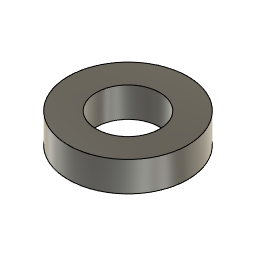
Question 4 Assembly (Autodesk Fusion 360 archive; units mm, degrees)
design "Spacer"
Autodesk Fusion 360 part; units mm, degrees
sketch "Sketch1" plane through (0, 0, 0) normal (0, 0, 1) x (1, 0, 0)
  circle A0 centre (0, 0) radius 8
  circle A1 centre (0, 0) radius 4.25
  dimension "d1" = 16
  dimension "d2" = 8.5
  constraint coincident A0.centre A1.centre
  measures "d1" diameter of A0
  measures "d2" diameter of A1
extrude "Extrude1" add sketch "Sketch1" along normal blind 4 makes body 1
copy_body "Body->Comp1" bodies 1 removing the originals makes body 2 in component "Component"
component "Component" placed x (1, 0, 0) y (0, 1, 0) z (0, 0, 1) at (0, 0, 0)

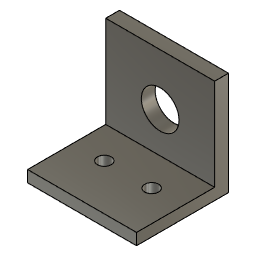
design "Support"
Autodesk Fusion 360 part; units mm, degrees
sketch "Sketch1" plane through (0, 0, 0) normal (0, 0, 1) x (1, 0, 0)
  line L0 (0, 0) -> (23.7, 0)
  line L1 (23.7, 0) -> (23.7, 20)
  line L2 (23.7, 20) -> (0, 20)
  line L3 (0, 20) -> (0, 0)
  line L4 (17, 0) -> (17, 10)
  circle A0 centre (17, 10) radius 1.5
  circle A1 centre (6.7, 10) radius 1.5
  dimension "d1" = 23.7
  dimension "d2" = 20
  dimension "d3" = 10
  dimension "d4" = 6.7
  dimension "d5" = 3
  dimension "d8" = -10.3
  dimension "d9" = 0
  constraint coincident L0.start L3.end
  constraint horizontal L0
  constraint perpendicular L0 L1
  constraint perpendicular L1 L2
  constraint perpendicular L0 L3
  constraint coincident L0 L4.start
  constraint perpendicular L0 L4
  constraint coincident L4.end A0.centre
  measures "d1" distance of L0.start L0.end
  measures "d2" distance of L0.end L1.end
  measures "d3" distance of L4.start L4.end
  measures "d4" distance of L1 L4
  measures "d5" diameter of A0
extrude "Extrude1" add sketch "Sketch1" along normal blind 2.5 makes body 1
sketch "Sketch2" plane through (0, 0, 2.5) normal (0, 0, 1) x (-1, 0, 0)
  circle A0 centre (-6.7, -10) radius 1.5
  circle A1 centre (-17, -10) radius 1.5
  line L0 (0, -20) -> (0, 0)
  line L1 (0, 0) -> (-23.7, 0)
  line L2 (-23.7, 0) -> (-23.7, -20)
  line L3 (-23.7, -20) -> (0, -20)
  line L4 (-23.7, -20) -> (-23.7, -17)
  line L5 (-23.7, -17) -> (0, -17)
  dimension "d12" = 3
  constraint coincident L2.end L3.start
  constraint perpendicular L3 L4
  constraint coincident L0 L5.end
  constraint perpendicular L0 L5
  measures "d12" distance of L2.end L4.end
extrude "Extrude2" add sketch "Sketch2" along normal blind 20 contours L0 L2 L3 L4 L5 bodies 1
sketch "Sketch3" plane through (0, 20, 0) normal (0, 1, 0) x (-1, 0, 0)
  line L0 (-23.7, 0) -> (0, 0)
  line L1 (0, 0) -> (0, 22.5)
  line L2 (0, 22.5) -> (-23.7, 22.5)
  line L3 (-23.7, 22.5) -> (-23.7, 0)
  line L4 (-23.7, 22.5) -> (0, 0)
  circle A0 centre (-11.85, 11.25) radius 4.1
  dimension "d15" = 8.2
  constraint coincident L2.end L3.start
  constraint coincident L0.end L1.start
  constraint midpoint L4 A0.centre
  measures "d15" diameter of A0
extrude "Extrude3" cut sketch "Sketch3" against normal blind 3 contours L4 A0 | L4 A0 bodies 1
copy_body "Body->Comp1" bodies 1 removing the originals makes body 2 in component "Component"
component "Component" placed x (1, 0, 0) y (0, 1, 0) z (0, 0, 1) at (0, 0, 0)

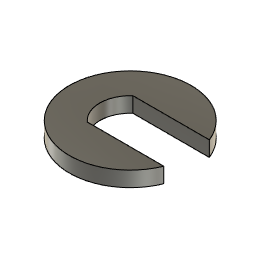
design "Collar"
Autodesk Fusion 360 part; units mm, degrees
sketch "Sketch1" plane through (0, 0, 0) normal (0, 0, 1) x (1, 0, 0)
  circle A0 centre (0, 0) radius 8
  circle A1 centre (0, 0) radius 4
  line L0 (11, -3) -> (-11, -3)
  line L1 (-11, -3) -> (-11, 3)
  line L2 (-11, 3) -> (11, 3)
  line L3 (11, 3) -> (11, -3)
  line L4 (11, -3) -> (-11, 3) construction
  line L5 (-11, -3) -> (11, 3) construction
  dimension "d1" = 16
  dimension "d2" = 8
  constraint coincident A0.centre A1.centre
  constraint horizontal L0
  constraint perpendicular L0 L1
  constraint parallel L0 L2
  constraint parallel L1 L3
  constraint coincident L4 A0.centre
  constraint coincident L5 A0.centre
  measures "d1" diameter of A0
  measures "d2" diameter of A1
extrude "Extrude1" add sketch "Sketch1" along normal blind 2 contours A0 A1 L2 | A0 A1 L0 | A0 A1 L0 L2 | A1 L2 | A1 L0 picked at (-6.3321, 2.0478) makes body 1
copy_body "Body->Comp1" bodies 1 removing the originals makes body 2 in component "Component"
component "Component" placed x (1, 0, 0) y (0, 1, 0) z (0, 0, 1) at (0, 0, 0)

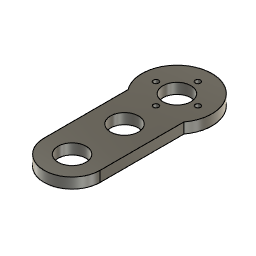
design "Input_Link"
Autodesk Fusion 360 part; units mm, degrees
sketch "Sketch1" plane through (0, 0, 0) normal (0, 0, 1) x (1, 0, 0)
  circle A0 centre (0, 0) radius 10
  circle A1 centre (0, 0) radius 4
  circle A2 centre (0, -15) radius 4
  circle A3 centre (0, -30) radius 4
  circle A4 centre (0, -30) radius 8
  line L0 (-8, -6) -> (-8, -30)
  line L1 (8, -6) -> (8, -30)
  line L2 (0, 0) -> (6, 0)
  circle A5 centre (6, 0) radius 0.75
  circle A6 centre (0, 6) radius 0.75
  circle A7 centre (-6, 0) radius 0.75
  circle A8 centre (0, -6) radius 0.75
  dimension "d1" = 20
  dimension "d2" = 8
  dimension "d5" = 0
  dimension "d6" = -30
  dimension "d7" = 16
  dimension "d9" = 8
  dimension "d12" = 6
  dimension "d14" = 360
  dimension "d15" = 1.5
  dimension "d16" = 8
  constraint coincident A0.centre A1.centre
  constraint concentric A3 A4
  constraint coincident A4 L0.end
  constraint coincident A0 L0.start
  constraint coincident A4 L1.end
  constraint coincident A0 L1.start
  constraint horizontal L2
  constraint coincident L2.end A5.centre
  measures "d1" diameter of A0
  measures "d2" diameter of A1
  measures "d7" diameter of A4
  measures "d9" distance of A3.centre L0
  measures "d12" distance of A0.centre L2.end
  measures "d15" diameter of A5
  measures "d16" distance of A3.centre L1
extrude "Extrude1" add sketch "Sketch1" along normal blind 3 makes body 1
copy_body "Body->Comp1" bodies 1 removing the originals makes body 2 in component "Component"
component "Component" placed x (1, 0, 0) y (0, 1, 0) z (0, 0, 1) at (0, 0, 0)

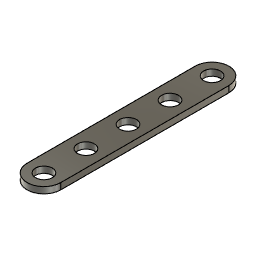
design "Coupler_Link"
Autodesk Fusion 360 part; units mm, degrees
sketch "Sketch1" plane through (0, 0, 0) normal (0, 0, 1) x (1, 0, 0)
  circle A0 centre (0, 0) radius 4
  circle A1 centre (0, 0) radius 8
  line L0 (-8, 0) -> (-8, -80)
  line L1 (8, 0) -> (8, -80)
  circle A2 centre (0, -80) radius 8
  circle A3 centre (0, -20) radius 4
  circle A4 centre (0, -40) radius 4
  circle A5 centre (0, -60) radius 4
  circle A6 centre (0, -80) radius 4
  dimension "d1" = 8
  dimension "d2" = 16
  dimension "d3" = 80
  dimension "d4" = 80
  dimension "d7" = 0
  dimension "d8" = -80
  dimension "d9" = 80
  dimension "d10" = 16
  constraint coincident A0.centre A1.centre
  constraint concentric A0 A1
  constraint coincident A1 L0.start
  constraint vertical L0
  constraint coincident A1 L1.start
  constraint coincident L1.end A2
  measures "d1" diameter of A0
  measures "d2" diameter of A1
  measures "d3" distance of L0.start L0.end
  measures "d4" distance of L1.start L1.end
  measures "d9" distance of A0.centre A2.centre
  measures "d10" distance of L0 L1
extrude "Extrude1" add sketch "Sketch1" along normal blind 3 makes body 1
copy_body "Body->Comp1" bodies 1 removing the originals makes body 2 in component "Component"
component "Component" placed x (1, 0, 0) y (0, 1, 0) z (0, 0, 1) at (0, 0, 0)

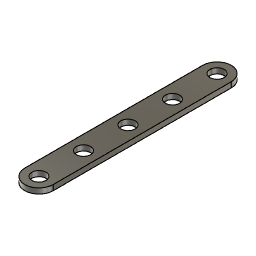
design "Output_Link"
Autodesk Fusion 360 part; units mm, degrees
sketch "Sketch1" plane through (0, 0, 0) normal (0, 0, 1) x (1, 0, 0)
  circle A0 centre (0, 0) radius 4
  circle A1 centre (0, 0) radius 8
  line L0 (-8, 0) -> (-8, -100)
  line L1 (8, 0) -> (8, -100)
  circle A2 centre (0, -100) radius 8
  circle A3 centre (0, -25) radius 4
  circle A4 centre (0, -50) radius 4
  circle A5 centre (0, -75) radius 4
  circle A6 centre (0, -100) radius 4
  dimension "d1" = 8
  dimension "d2" = 16
  dimension "d3" = 100
  dimension "d4" = 100
  dimension "d7" = 0
  dimension "d8" = -100
  constraint coincident A0.centre A1.centre
  constraint coincident A1 L0.start
  constraint tangent A1 L0
  constraint coincident A1 L1.start
  constraint coincident L1.end A2
  measures "d1" diameter of A0
  measures "d2" diameter of A1
  measures "d3" distance of L0.start L0.end
  measures "d4" distance of L1.start L1.end
extrude "Extrude1" add sketch "Sketch1" along normal blind 3 makes body 1
copy_body "Body->Comp1" bodies 1 removing the originals makes body 2 in component "Component"
component "Component" placed x (1, 0, 0) y (0, 1, 0) z (0, 0, 1) at (0, 0, 0)

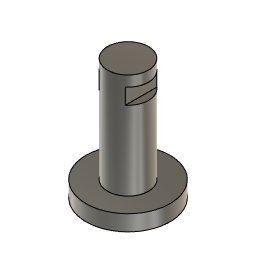
design "Pin_Joint"
Autodesk Fusion 360 part; units mm, degrees
sketch "Sketch1" plane through (0, 0, 0) normal (0, 0, 1) x (1, 0, 0)
  circle A0 centre (0, 0) radius 8
  dimension "d1" = 16
  constraint coincident A0.centre origin
  measures "d1" diameter of A0
extrude "Extrude1" add sketch "Sketch1" along normal blind 3 makes body 1
sketch "Sketch2" plane through (0, 0, 3) normal (0, 0, 1) x (-1, 0, 0)
  circle A0 centre (0, 0) radius 8
  circle A1 centre (0, 0) radius 3.9
  dimension "d4" = 7.8
  constraint concentric A0 A1
  measures "d4" diameter of A1
extrude "Extrude2" add sketch "Sketch2" along normal blind 15 contours A1 bodies 1
sketch "Sketch3" plane through (0, 0, 18) normal (0, 0, 1) x (-1, 0, 0)
  circle A0 centre (0, 0) radius 3.9
  line L0 (-2.5, -6.25) -> (2.5, -6.25)
  line L1 (2.5, -6.25) -> (2.5, 6.25)
  line L2 (2.5, 6.25) -> (-2.5, 6.25)
  line L3 (-2.5, 6.25) -> (-2.5, -6.25)
  line L4 (-2.5, -6.25) -> (2.5, 6.25) construction
  line L5 (2.5, -6.25) -> (-2.5, 6.25) construction
  dimension "d12" = 5
  constraint horizontal L0
  constraint perpendicular L0 L1
  constraint parallel L0 L2
  constraint parallel L1 L3
  constraint coincident L4 A0.centre
  constraint coincident L5 A0.centre
  constraint coincident A0.centre origin
  measures "d12" distance of L1 L3
extrude "Extrude3" add sketch "Sketch3" along normal blind 3 contours A0 L1 L3 bodies 1
sketch "Sketch4" plane through (0, 0, 21) normal (0, 0, 1) x (-1, 0, 0)
  arc A0 (2.5, 2.9933) -> (-2.5, 2.9933) centre (0, 0) ccw
  line L0 (-2.5, 2.9933) -> (-2.5, -2.9933)
  arc A1 (-2.5, -2.9933) -> (2.5, -2.9933) centre (0, 0) ccw
  line L1 (2.5, -2.9933) -> (2.5, 2.9933)
  circle A2 centre (0, 0) radius 3.9
  dimension "d9" = 7.8
  constraint concentric A0 A2
  measures "d9" diameter of A2
extrude "Extrude4" add sketch "Sketch4" along normal blind 2 bodies 1
copy_body "Body->Comp1" bodies 1 removing the originals makes body 2 in component "Component"
component "Component" placed x (1, 0, 0) y (0, 1, 0) z (0, 0, 1) at (0, 0, 0)

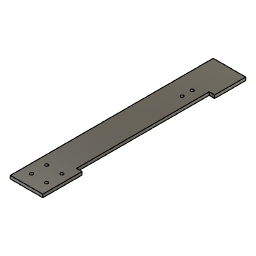
design "Base_Link"
Autodesk Fusion 360 part; units mm, degrees
sketch "Sketch3" plane through (0, 0, 0) normal (0, 0, 1) x (1, 0, 0)
  line L0 (0, 0) -> (0, 200)
  line L1 (0, 200) -> (32.04, 200)
  line L2 (32.04, 200) -> (32.04, 169.36)
  line L3 (32.04, 169.36) -> (26.64, 169.36)
  line L4 (0, 0) -> (32.04, 0)
  line L5 (32.04, 0) -> (32.04, 38.69)
  line L6 (32.04, 38.69) -> (26.64, 38.69)
  line L7 (26.64, 38.69) -> (26.64, 169.36)
  circle A0 centre (9.04, 11.845) radius 1.5
  circle A1 centre (24.04, 11.845) radius 1.5
  circle A2 centre (9.04, 26.845) radius 1.5
  circle A3 centre (24.04, 26.845) radius 1.5
  circle A4 centre (17.04, 162.36) radius 1.5
  circle A5 centre (17.04, 152.36) radius 1.5
  dimension "d1" = 200
  dimension "d2" = 32.04
  dimension "d3" = 30.64
  dimension "d4" = 5.4
  dimension "d5" = 32.04
  dimension "d6" = 38.69
  dimension "d7" = 5.4
  dimension "d11" = 3
  dimension "d14" = 15
  dimension "d15" = 15
  dimension "d16" = 9.04
  dimension "d17" = 11.845
  dimension "d20" = 3
  dimension "d21" = 9.6
  dimension "d22" = 37.64
  dimension "d25" = 0
  dimension "d26" = -10
  constraint coincident L0.start L4.start
  constraint vertical L0
  constraint perpendicular L0 L1
  constraint perpendicular L1 L2
  constraint perpendicular L2 L3
  constraint perpendicular L0 L4
  constraint perpendicular L4 L5
  constraint perpendicular L5 L6
  measures "d1" distance of L0.start L0.end
  measures "d2" distance of L0.end L1.end
  measures "d3" distance of L1.end L2.end
  measures "d4" distance of L2.end L3.end
  measures "d5" distance of L0.start L4.end
  measures "d6" distance of L4.end L5.end
  measures "d7" distance of L5.end L6.end
  measures "d11" diameter of A0
  measures "d16" distance of L0 A0.centre
  measures "d17" distance of L4 A0.centre
  measures "d20" diameter of A4
  measures "d21" distance of L7 A4.centre
  measures "d22" distance of L1 A4.centre
extrude "Extrude1" add sketch "Sketch3" along normal blind 3 makes body 1
copy_body "Body->Comp1" bodies 1 removing the originals makes body 2 in component "Component"
component "Component" placed x (1, 0, 0) y (0, 1, 0) z (0, 0, 1) at (0, 0, 0)

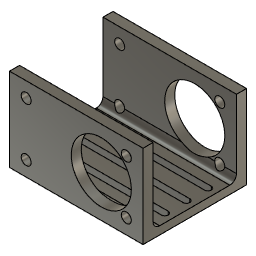
design "Motor_Holder"
Autodesk Fusion 360 part; units mm, degrees
sketch "Sketch2" plane through (0, 0, 0) normal (1, 0, 0) x (0, 1, 0)
  line L0 (0, 0) -> (31, 0)
  line L1 (0, 0) -> (0, 25)
  line L2 (31, 0) -> (31, 25)
  line L3 (0, 25) -> (3, 25)
  line L4 (31, 0) -> (31, 2.4)
  line L5 (31, 2.4) -> (0, 2.4)
  line L6 (3, 25) -> (3, 2.4)
  line L7 (31, 25) -> (28, 25)
  line L8 (28, 25) -> (28, 2.4)
  line L9 (3, 2.4) -> (5, 2.4)
  line L10 (3, 4.4) -> (3, 2.4)
  circle A0 centre (5, 4.4) radius 2
  line L11 (28, 2.4) -> (26, 2.4)
  line L12 (28, 4.4) -> (28, 2.4)
  circle A1 centre (26, 4.4) radius 2
  dimension "d4" = 31
  dimension "d5" = 2.4
  dimension "d6" = 3
  dimension "d7" = 22.6
  dimension "d8" = 3
  dimension "d9" = 22.6
  dimension "d10" = 2
  dimension "d11" = 2
  dimension "d12" = 2
  constraint coincident L0.start L1.start
  constraint horizontal L0
  constraint perpendicular L0 L1
  constraint perpendicular L0 L2
  constraint perpendicular L1 L3
  constraint perpendicular L0 L4
  constraint coincident L1 L5.end
  constraint perpendicular L1 L5
  constraint coincident L5 L6.end
  constraint perpendicular L5 L6
  constraint perpendicular L2 L7
  constraint coincident L5 L8.end
  constraint perpendicular L5 L8
  constraint horizontal L9
  constraint vertical L10
  constraint coincident L9.end A0
  constraint horizontal L11
  constraint vertical L12
  constraint coincident L11.end A1
  measures "d4" distance of L0.start L0.end
  measures "d5" distance of L0.end L4.end
  measures "d6" distance of L1.end L3.end
  measures "d7" distance of L3 L5
  measures "d8" distance of L2.end L7.end
  measures "d9" distance of L5 L7
  measures "d10" distance of L6.end L10.start
  measures "d11" distance of L8.end L11.end
  measures "d12" distance of L8.end L12.start
extrude "Extrude1" add sketch "Sketch2" along normal blind 40 contours L0 L1 L2 L4 L5 L9 L11 | L1 L3 L5 L6 L10 | L2 L5 L7 L8 L12 | L5 L6 L9 L10 A0 | L5 L8 L11 L12 A1 makes body 1
sketch "Sketch3" plane through (0, 0, 0) normal (0, 0, -1) x (1, 0, 0)
  line L0 (0, 0) -> (0, -31)
  line L1 (0, -31) -> (40, -31)
  line L2 (40, -31) -> (40, 0)
  line L3 (40, 0) -> (0, 0)
  line L4 (0, 0) -> (2.5, 0)
  circle A0 centre (2.5, -9.04) radius 1
  circle A1 centre (37.5, -9.04) radius 1
  line L5 (37.5, -8.04) -> (2.5, -8.04)
  line L6 (2.5, -10.04) -> (37.5, -10.04)
  circle A2 centre (2.5, -15.5) radius 1
  line L7 (37.5, -14.5) -> (2.5, -14.5)
  line L8 (2.5, -16.5) -> (37.5, -16.5)
  circle A3 centre (37.5, -15.5) radius 1
  circle A4 centre (2.5, -21.96) radius 1
  line L9 (37.5, -20.96) -> (2.5, -20.96)
  line L10 (2.5, -22.96) -> (37.5, -22.96)
  circle A5 centre (37.5, -21.96) radius 1
  dimension "d15" = 2.5
  dimension "d16" = 9.04
  dimension "d17" = 2
  dimension "d20" = 35
  dimension "d21" = 0
  dimension "d24" = 0
  dimension "d25" = -12.92
  constraint coincident L0.start L3.end
  constraint perpendicular L0 L4
  constraint coincident A1 L5.start
  constraint coincident A0 L5.end
  constraint coincident A0 L6.start
  constraint coincident A1 L6.end
  constraint tangent A1 L6
  measures "d15" distance of L0.start L4.end
  measures "d16" distance of L4.end A0.centre
  measures "d17" diameter of A0
extrude "Extrude2" cut sketch "Sketch3" against normal blind 2.4 contours A0 | A0 A1 L5 L6 | A1 | A2 | A2 L7 L8 A3 | A3 | A4 | A4 L9 L10 A5 | A5 bodies 1
sketch "Sketch4" plane through (0, 31, 0) normal (0, 1, 0) x (-1, 0, 0)
  line L0 (0, 0) -> (0, 25)
  line L1 (0, 25) -> (-40, 25)
  line L2 (-40, 25) -> (-40, 0)
  line L3 (-40, 0) -> (0, 0)
  line L4 (-35, 25) -> (-35, 20.5)
  circle A0 centre (-35, 20.5) radius 1.5
  circle A1 centre (-5, 20.5) radius 1.5
  circle A2 centre (-35, 4.5) radius 1.5
  circle A3 centre (-5, 4.5) radius 1.5
  line L5 (-40, 0) -> (-27.5, 0)
  line L6 (-27.5, 0) -> (-27.5, 12.5)
  line L7 (-27.5, 12.5) -> (-40, 12.5)
  line L8 (-40, 12.5) -> (-40, 0)
  circle A4 centre (-27.5, 12.5) radius 9
  dimension "d29" = 4.5
  dimension "d30" = 5
  dimension "d31" = 3
  dimension "d34" = 30
  dimension "d35" = -16
  dimension "d36" = 12.5
  dimension "d37" = 12.5
  dimension "d38" = 18
  constraint coincident L1 L4.start
  constraint perpendicular L1 L4
  constraint coincident L4.end A0.centre
  constraint horizontal L5
  constraint vertical L6
  constraint horizontal L7
  constraint vertical L8
  constraint coincident L2.end L3.start
  constraint coincident L6.end L7.start
  measures "d29" distance of L4.start L4.end
  measures "d30" distance of L2 L4
  measures "d31" diameter of A0
  measures "d36" distance of L2.end L5.end
  measures "d37" distance of L2.end L7.end
  measures "d38" diameter of A4
extrude "Extrude3" cut sketch "Sketch4" against normal blind 31 contours L6 L7 A4 | L6 L7 A4 | A0 | A1 | A2 | A3 bodies 1
copy_body "Body->Comp1" bodies 1 removing the originals makes body 2 in component "Component"
component "Component" placed x (1, 0, 0) y (0, 1, 0) z (0, 0, 1) at (0, 0, 0)
